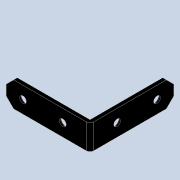
# Autodesk Inventor part: 90 deg Shelf 4 Hole Bracket
Saved by Autodesk Inventor 2022 (Build 260153000, 153)
## iProperties
Created: 2021-12-19
Part Number: 90 deg Shelf 4 Hole Bracket
Material: Generic
Document SubType Name: Modeling
Designer: Coy
Density: 1 g/cm^3
Appearance: Anodized - Black
Author: Coy
Autodesk Inventor part; units mm, degrees
ref_plane "YZ Plane" through (0, 0, 0) normal (1, 0, 0) x (0, 1, 0)
ref_plane "XZ Plane" through (0, 0, 0) normal (0, 1, 0) x (-1, 0, 0)
ref_plane "XY Plane" through (0, 0, 0) normal (0, 0, 1) x (1, 0, 0)
sketch "Sketch1" plane through (0, 0, 0) normal (0, 1, 0) x (-1, 0, 0)
  line L0 (0, 0) -> (0, 67)
  line L1 (0, 67) -> (67, 67)
  line L2 (67, 64) -> (3, 64)
  line L3 (3, 64) -> (3, 0)
  line L4 (67, 67) -> (67, 64)
  line L5 (3, 0) -> (0, 0)
  dimension "d0" = 67
  dimension "d1" = 67
  dimension "d2" = 3
  constraints: 12 end point, 3 perpendicular, 2 vertical, 1 other
  measures "d0" distance of L0.start L0.end
  measures "d1" distance of L0.end L1.end
  measures "d2" distance between parallel lines of L1 L2
extrude "Extrusion1" add sketch "Sketch1" along normal blind 20
sketch "Sketch2" plane through (-3, 0, 64) normal (0, 0, -1) x (-1, 0, 0)
  line L0 (64, 0) -> (64, 20) construction
  line L1 (64, 10) -> (0, 10) construction
  line L2 (0, 0) -> (0, 20) construction
  circle A0 centre (50.5, 10) radius 2.65
  circle A1 centre (18.7, 10) radius 2.65
  point P0 (-3, 0)
  dimension "d5" = 5.3
  dimension "d6" = 5.3
  dimension "d7" = 13.5
  dimension "d8" = 31.8
  constraints: 2 centre point, 2 end point, 2 midpoint, 2 point on line
  measures "d5" diameter of A0
  measures "d6" diameter of A1
  measures "d7" distance from line of L0 A0.centre
  measures "d8" distance of A1.centre A0.centre
extrude "Extrusion2" cut sketch "Sketch2" against normal up to next
sketch "Sketch3" plane through (-3, 0, 0) normal (-1, 0, 0) x (0, 0, 1)
  line L0 (0, 0) -> (0, 20) construction
  line L1 (0, 10) -> (64, 10) construction
  line L2 (64, 0) -> (64, 20) construction
  circle A0 centre (13.5, 10) radius 2.65
  circle A1 centre (45.3, 10) radius 2.65
  dimension "d11" = 5.3
  dimension "d12" = 5.3
  dimension "d13" = 13.5
  dimension "d14" = 31.8
  constraints: 2 centre point, 2 end point, 2 midpoint, 2 point on line
  measures "d11" diameter of A0
  measures "d12" diameter of A1
  measures "d13" distance from line of L0 A0.centre
  measures "d14" distance of A1.centre A0.centre
extrude "Extrusion3" cut sketch "Sketch3" against normal up to next
chamfer "Chamfer1" distance 2 angle 45 4 edges at (-50.85, 10, 64) (-19.05, 10, 64) (-3, 10, 42.65) (-3, 10, 10.85)
chamfer "Chamfer2" distance 6 angle 45 4 edges at (-67, 0, 65.5) (-67, 20, 65.5) (-1.5, 0, 0) (-1.5, 20, 0)
fillet "Fillet1" radius 3 1 edges at (0, 10, 67)
equation "\"d1\" = d0"
equation "\"d6\" = d5"
equation "\"d12\" = d11"
body "Solid1"
